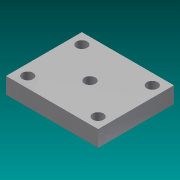
# Autodesk Inventor part: dudukan u bolt
Saved by Autodesk Inventor 2014 SP2 (Build 180246200, 246)
## iProperties
Created: 2019-07-17
Part Number: dudukan u bolt
Material: Steel, Mild
Document SubType Name: Modeling
Designer: USER PC
Density: 7.86 g/cm^3
Appearance: Steel
Author: USER PC
Autodesk Inventor part; units mm, degrees
ref_plane "YZ Plane" through (0, 0, 0) normal (1, 0, 0) x (0, 1, 0)
ref_plane "XZ Plane" through (0, 0, 0) normal (0, 1, 0) x (-1, 0, 0)
ref_plane "XY Plane" through (0, 0, 0) normal (0, 0, 1) x (1, 0, 0)
sketch "Sketch1" plane through (0, 0, 0) normal (0, 0, 1) x (1, 0, 0)
  circle A0 centre (0, 0) radius 5
  line L0 (-42.5, 35) -> (42.5, 35)
  line L1 (42.5, 35) -> (42.5, -35)
  line L2 (42.5, -35) -> (-42.5, -35)
  line L3 (-42.5, -35) -> (-42.5, 35)
  line L4 (42.5, 35) -> (-42.5, -35) construction
  line L5 (0, 15) -> (0, -15)
  circle A1 centre (-32.5, 25) radius 5
  circle A2 centre (32.5, 25) radius 5
  circle A3 centre (-32.5, -25) radius 5
  circle A4 centre (32.5, -25) radius 5
  dimension "d0" = 10
  dimension "d1" = 70
  dimension "d2" = 85
  dimension "d3" = 15
  dimension "d4" = 30
  dimension "d5" = 10
  dimension "d6" = 10
  dimension "d7" = 10
  dimension "d8" = 10
  dimension "d11" = 65
  constraints: 12 end point, 5 centre point, 2 parallel, 1 coincident, 1 horizontal, 1 midpoint, 1 perpendicular
  measures "d0" diameter of A0
  measures "d1" distance of L0.end L1.end
  measures "d2" distance of L1.end L2.end
  measures "d3" distance of A0.centre L5.start
  measures "d4" distance of L5.start L5.end
  measures "d5" diameter of A1
  measures "d6" distance from line of A1.centre L3
  measures "d7" distance from line of L0 A1.centre
  measures "d8" distance from line of L1 A2.centre
  measures "d11" distance of A1.centre A2.centre
extrude "Extrusion1" add sketch "Sketch1" along normal blind 15
body "Solid1"
